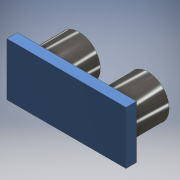
# Autodesk Inventor part: HC-SR04
Saved by Autodesk Inventor 2016 (Build 200138000, 138)
## iProperties
Created: 2016-04-26
Part Number: HC-SR04
Material: Generic
Document SubType Name: Modeling
Designer: Owner
Density: 1 g/cm^3
Appearance: Default
Author: Owner
Autodesk Inventor part; units mm, degrees
ref_plane "YZ Plane" through (0, 0, 0) normal (1, 0, 0) x (0, 1, 0)
ref_plane "XZ Plane" through (0, 0, 0) normal (0, 1, 0) x (-1, 0, 0)
ref_plane "XY Plane" through (0, 0, 0) normal (0, 0, 1) x (1, 0, 0)
sketch "Sketch1" plane through (0, 0, 0) normal (0, 1, 0) x (-1, 0, 0)
  line L0 (0, 0) -> (45, 0)
  line L1 (45, 0) -> (45, -20)
  line L2 (45, -20) -> (0, -20)
  line L3 (0, -20) -> (0, 0)
  dimension "d0" = 45
  dimension "d1" = 20
  constraints: 8 end point, 2 parallel, 1 horizontal, 1 perpendicular
  measures "d0" distance of L1.end L2.end
  measures "d1" distance of L2.end L0.start
extrude "Extrusion1" add sketch "Sketch1" along normal blind 4
sketch "Sketch2" plane through (0, 4, 0) normal (0, 1, 0) x (1, 0, 0)
  line L0 (0, 0) -> (0, 20) projected
  line L1 (-45, 20) -> (-45, 0) projected
  line L2 (-45, 10) -> (-35.5, 10)
  line L3 (0, 10) -> (-9.5, 10)
  circle A0 centre (-9.5, 10) radius 8
  circle A1 centre (-35.5, 10) radius 8
  line L4 (-35.5, 10) -> (-9.5, 10)
  dimension "d4" = 9.5
  dimension "d5" = 9.5
  dimension "d6" = 16
  dimension "d7" = 16
  dimension "d8" = 26
  constraints: 6 end point, 3 horizontal, 2 centre point, 2 coincident, 2 midpoint
  measures "d4" distance of L2.start L2.end
  measures "d5" distance of L3.start L3.end
  measures "d6" diameter of A0
  measures "d7" diameter of A1
  measures "d8" distance of L4.start L4.end
extrude "Extrusion2" add sketch "Sketch2" along normal blind 13.8
body "Solid1"
